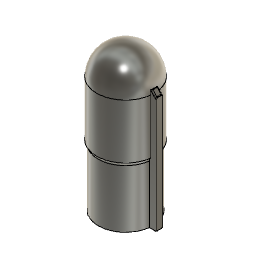
Dr.J Adapter v3 (Autodesk Fusion 360 design; units mm, degrees)
Autodesk Fusion 360 part; units mm, degrees
sketch "Sketch1" plane through (0, 0, 0) normal (0, 0, 1) x (1, 0, 0)
  circle A0 centre (0, 0) radius 12.5
  dimension "d1" = 25
  constraint coincident A0.centre origin
  measures "d1" diameter of A0
extrude "Extrude1" add sketch "Sketch1" along normal blind 28
sketch "Sketch2" plane through (0, 0, 28) normal (0, 0, 1) x (-1, 0, 0)
  circle A0 centre (0, 0) radius 12.5
  circle A1 centre (0, 0) radius 13.25
  dimension "d4" = 26.5
  constraint coincident A0.centre A1.centre
  measures "d4" diameter of A1
extrude "Extrude2" add sketch "Sketch2" along normal blind 25 contours A0 | A1
sphere "SpherePrimitive1" add diameter 26.5 placed x (-1, 0, 0) y (0, -1, 0) z (0, 0, 1) at (0, 0, 53)
sketch "Sketch4" plane through (0, 0, 0) normal (0, 0, -1) x (1, 0, 0)
  circle A0 centre (0, 0) radius 12.5
  circle A1 centre (0, 0) radius 2.75
  dimension "d8" = 5.5
  constraint coincident A0.centre A1.centre
  measures "d8" diameter of A1
extrude "Extrude3" cut sketch "Sketch4" against normal blind 31 contours A1
fillet "Fillet1" radius 2 1 edges at (-11.6541, -4.5202, 28)
ref_plane "WorkPlane1" through (12.5, 0, 13.0606) normal (1, 0, 0) x (0, -1, 0)
sketch "Sketch5" plane through (12.5, 0, 0) normal (1, 0, 0) x (0, 1, 0)
  line L0 (-1.5, 0) -> (1.5, 0)
  line L1 (1.5, 0) -> (1.5, 55)
  line L2 (1.5, 55) -> (-1.5, 55)
  line L3 (-1.5, 55) -> (-1.5, 0)
  dimension "d14" = 3
  dimension "d15" = 55
  constraint horizontal L0
  constraint vertical L1
  constraint horizontal L2
  constraint vertical L3
  constraint midpoint L0 origin
  measures "d14" distance of L0.start L0.end
  measures "d15" distance of L0.start L2.end
extrude "Extrude4" add sketch "Sketch5" along normal blind 3
chamfer "Chamfer1" distance 2 angle 45 1 edges at (15.5, 0, 55)
fillet "Fillet2" radius 0.5 3 edges at (15.5, 0, 53) (14.5, -1.5, 54) (14.5, 1.5, 54)
